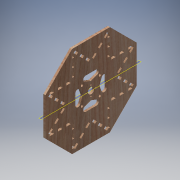
# Autodesk Inventor part: OctBase
Saved by Autodesk Inventor 2019 (Build 230136000, 136)
## iProperties
Created: 2019-01-14
Part Number: OctBase
Material: Wood (Birch)
Document SubType Name: Modeling
Designer: nxgam
Density: 0.55 g/cm^3
Appearance: Birch - Natural Polished
Author: nxgam
Autodesk Inventor part; units mm, degrees
ref_plane "YZ Plane" through (0, 0, 0) normal (1, 0, 0) x (0, 1, 0)
ref_plane "XZ Plane" through (0, 0, 0) normal (0, 1, 0) x (-1, 0, 0)
ref_plane "XY Plane" through (0, 0, 0) normal (0, 0, 1) x (1, 0, 0)
sketch "Sketch1" plane through (0, 0, 0) normal (1, 0, 0) x (0, 1, 0)
  line L0 (-110.3778, -45.72) -> (-110.3778, 45.72)
  line L1 (-110.3778, 45.72) -> (-45.72, 110.3778)
  line L2 (-45.72, 110.3778) -> (45.72, 110.3778)
  line L3 (45.72, 110.3778) -> (110.3778, 45.72)
  line L4 (110.3778, 45.72) -> (110.3778, -45.72)
  line L5 (110.3778, -45.72) -> (45.72, -110.3778)
  line L6 (45.72, -110.3778) -> (-45.72, -110.3778)
  line L7 (-45.72, -110.3778) -> (-110.3778, -45.72)
  point P0 (0, 0)
  point P1 (0, 0)
  dimension "d0" = 91.44
  constraints: 16 end point, 1 coincident, 1 horizontal, 17 other
  measures "d0" distance of L3.end L4.end
extrude "Extrusion1" add sketch "Sketch1" along normal blind 5.08
sketch "Sketch2" plane through (5.08, 0, 0) normal (1, 0, 0) x (0, 0, -1)
  line L0 (-45.72, 59.5778) -> (-40.64, 59.5778)
  line L1 (-40.64, 59.5778) -> (-40.64, 49.4178)
  line L2 (-40.64, 49.4178) -> (-45.72, 49.4178)
  line L3 (-45.72, 49.4178) -> (-45.72, 59.5778)
  line L4 (-45.72, 79.8978) -> (-40.64, 79.8978)
  line L5 (-40.64, 79.8978) -> (-40.64, 69.7378)
  line L6 (-40.64, 69.7378) -> (-45.72, 69.7378)
  line L7 (-45.72, 69.7378) -> (-45.72, 79.8978)
  line L8 (-45.72, 100.2178) -> (-40.64, 100.2178)
  line L9 (-40.64, 100.2178) -> (-40.64, 90.0578)
  line L10 (-40.64, 90.0578) -> (-45.72, 90.0578)
  line L11 (-45.72, 90.0578) -> (-45.72, 100.2178)
  line L12 (-40.64, 110.3778) -> (-45.72, 110.3778)
  line L13 (-45.72, 110.3778) -> (-45.72, 120.5378)
  line L14 (-45.72, 120.5378) -> (-40.64, 120.5378)
  line L15 (-40.64, 120.5378) -> (-40.64, 110.3778)
  line L16 (-45.72, 130.6978) -> (-45.72, 140.8578)
  line L17 (-45.72, 140.8578) -> (-40.64, 140.8578)
  line L18 (-40.64, 140.8578) -> (-40.64, 130.6978)
  line L19 (-40.64, 130.6978) -> (-45.72, 130.6978)
  line L20 (-45.72, 151.0178) -> (-45.72, 161.1778)
  line L21 (-45.72, 161.1778) -> (-40.64, 161.1778)
  line L22 (-40.64, 161.1778) -> (-40.64, 151.0178)
  line L23 (-40.64, 151.0178) -> (-45.72, 151.0178)
  line L24 (-45.72, 171.3378) -> (-45.72, 181.4978)
  line L25 (-45.72, 181.4978) -> (-40.64, 181.4978)
  line L26 (-40.64, 181.4978) -> (-40.64, 171.3378)
  line L27 (-40.64, 171.3378) -> (-45.72, 171.3378)
  line L28 (-45.72, 191.6578) -> (-45.72, 201.8178)
  line L29 (-45.72, 201.8178) -> (-40.64, 201.8178)
  line L30 (-40.64, 201.8178) -> (-40.64, 191.6578)
  line L31 (-40.64, 191.6578) -> (-45.72, 191.6578)
  line L32 (-45.72, 211.9778) -> (-45.72, 222.1378)
  line L33 (-45.72, 222.1378) -> (-40.64, 222.1378)
  line L34 (-40.64, 222.1378) -> (-40.64, 211.9778)
  line L35 (-40.64, 211.9778) -> (-45.72, 211.9778)
  line L36 (-45.72, 232.2978) -> (-45.72, 242.4578)
  line L37 (-45.72, 242.4578) -> (-40.64, 242.4578)
  line L38 (-40.64, 242.4578) -> (-40.64, 232.2978)
  line L39 (-40.64, 232.2978) -> (-45.72, 232.2978)
  line L40 (-45.72, 252.6178) -> (-45.72, 262.7778)
  line L41 (-45.72, 262.7778) -> (-40.64, 262.7778)
  line L42 (-40.64, 262.7778) -> (-40.64, 252.6178)
  line L43 (-40.64, 252.6178) -> (-45.72, 252.6178)
  line L44 (-45.72, 272.9378) -> (-45.72, 283.0978)
  line L45 (-45.72, 283.0978) -> (-40.64, 283.0978)
  line L46 (-40.64, 283.0978) -> (-40.64, 272.9378)
  line L47 (-40.64, 272.9378) -> (-45.72, 272.9378)
  line L48 (-45.72, 293.2578) -> (-45.72, 303.4178)
  line L49 (-45.72, 303.4178) -> (-40.64, 303.4178)
  line L50 (-40.64, 303.4178) -> (-40.64, 293.2578)
  line L51 (-40.64, 293.2578) -> (-45.72, 293.2578)
  line L52 (-45.72, 313.5778) -> (-45.72, 323.7378)
  line L53 (-45.72, 323.7378) -> (-40.64, 323.7378)
  line L54 (-40.64, 323.7378) -> (-40.64, 313.5778)
  line L55 (-40.64, 313.5778) -> (-45.72, 313.5778)
  line L56 (-45.72, 333.8978) -> (-45.72, 344.0578)
  line L57 (-45.72, 344.0578) -> (-40.64, 344.0578)
  line L58 (-40.64, 344.0578) -> (-40.64, 333.8978)
  line L59 (-40.64, 333.8978) -> (-45.72, 333.8978)
  line L60 (-45.72, 354.2178) -> (-45.72, 364.3778)
  line L61 (-45.72, 364.3778) -> (-40.64, 364.3778)
  line L62 (-40.64, 364.3778) -> (-40.64, 354.2178)
  line L63 (-40.64, 354.2178) -> (-45.72, 354.2178)
  line L64 (-45.72, 374.5378) -> (-45.72, 384.6978)
  line L65 (-45.72, 384.6978) -> (-40.64, 384.6978)
  line L66 (-40.64, 384.6978) -> (-40.64, 374.5378)
  line L67 (-40.64, 374.5378) -> (-45.72, 374.5378)
  line L68 (-45.72, 394.8578) -> (-45.72, 405.0178)
  line L69 (-45.72, 405.0178) -> (-40.64, 405.0178)
  line L70 (-40.64, 405.0178) -> (-40.64, 394.8578)
  line L71 (-40.64, 394.8578) -> (-45.72, 394.8578)
  line L72 (-45.72, 415.1778) -> (-45.72, 425.3378)
  line L73 (-45.72, 425.3378) -> (-40.64, 425.3378)
  line L74 (-40.64, 425.3378) -> (-40.64, 415.1778)
  line L75 (-40.64, 415.1778) -> (-45.72, 415.1778)
  line L76 (-45.72, 435.4978) -> (-45.72, 473.3735)
  line L77 (-45.72, 473.3735) -> (-40.64, 473.3735)
  line L78 (-40.64, 473.3735) -> (-40.64, 435.4978)
  line L79 (-40.64, 435.4978) -> (-45.72, 435.4978)
  line L80 (40.64, 59.5778) -> (45.72, 59.5778)
  line L81 (45.72, 59.5778) -> (45.72, 49.4178)
  line L82 (45.72, 49.4178) -> (40.64, 49.4178)
  line L83 (40.64, 49.4178) -> (40.64, 59.5778)
  line L84 (40.64, 79.8978) -> (45.72, 79.8978)
  line L85 (45.72, 79.8978) -> (45.72, 69.7378)
  line L86 (45.72, 69.7378) -> (40.64, 69.7378)
  line L87 (40.64, 69.7378) -> (40.64, 79.8978)
  line L88 (40.64, 100.2178) -> (45.72, 100.2178)
  line L89 (45.72, 100.2178) -> (45.72, 90.0578)
  line L90 (45.72, 90.0578) -> (40.64, 90.0578)
  line L91 (40.64, 90.0578) -> (40.64, 100.2178)
  line L92 (45.72, 110.3778) -> (40.64, 110.3778)
  line L93 (40.64, 110.3778) -> (40.64, 120.5378)
  line L94 (40.64, 120.5378) -> (45.72, 120.5378)
  line L95 (45.72, 120.5378) -> (45.72, 110.3778)
  line L96 (40.64, 130.6978) -> (40.64, 140.8578)
  line L97 (40.64, 140.8578) -> (45.72, 140.8578)
  line L98 (45.72, 140.8578) -> (45.72, 130.6978)
  line L99 (45.72, 130.6978) -> (40.64, 130.6978)
  line L100 (40.64, 151.0178) -> (40.64, 161.1778)
  line L101 (40.64, 161.1778) -> (45.72, 161.1778)
  line L102 (45.72, 161.1778) -> (45.72, 151.0178)
  line L103 (45.72, 151.0178) -> (40.64, 151.0178)
  line L104 (40.64, 171.3378) -> (40.64, 181.4978)
  line L105 (40.64, 181.4978) -> (45.72, 181.4978)
  line L106 (45.72, 181.4978) -> (45.72, 171.3378)
  line L107 (45.72, 171.3378) -> (40.64, 171.3378)
  line L108 (40.64, 191.6578) -> (40.64, 201.8178)
  line L109 (40.64, 201.8178) -> (45.72, 201.8178)
  line L110 (45.72, 201.8178) -> (45.72, 191.6578)
  line L111 (45.72, 191.6578) -> (40.64, 191.6578)
  line L112 (40.64, 211.9778) -> (40.64, 222.1378)
  line L113 (40.64, 222.1378) -> (45.72, 222.1378)
  line L114 (45.72, 222.1378) -> (45.72, 211.9778)
  line L115 (45.72, 211.9778) -> (40.64, 211.9778)
  line L116 (40.64, 232.2978) -> (40.64, 242.4578)
  line L117 (40.64, 242.4578) -> (45.72, 242.4578)
  line L118 (45.72, 242.4578) -> (45.72, 232.2978)
  line L119 (45.72, 232.2978) -> (40.64, 232.2978)
  line L120 (40.64, 252.6178) -> (40.64, 262.7778)
  line L121 (40.64, 262.7778) -> (45.72, 262.7778)
  line L122 (45.72, 262.7778) -> (45.72, 252.6178)
  line L123 (45.72, 252.6178) -> (40.64, 252.6178)
  line L124 (40.64, 272.9378) -> (40.64, 283.0978)
  line L125 (40.64, 283.0978) -> (45.72, 283.0978)
  line L126 (45.72, 283.0978) -> (45.72, 272.9378)
  line L127 (45.72, 272.9378) -> (40.64, 272.9378)
  line L128 (40.64, 293.2578) -> (40.64, 303.4178)
  line L129 (40.64, 303.4178) -> (45.72, 303.4178)
  line L130 (45.72, 303.4178) -> (45.72, 293.2578)
  line L131 (45.72, 293.2578) -> (40.64, 293.2578)
  line L132 (40.64, 313.5778) -> (40.64, 323.7378)
  line L133 (40.64, 323.7378) -> (45.72, 323.7378)
  line L134 (45.72, 323.7378) -> (45.72, 313.5778)
  line L135 (45.72, 313.5778) -> (40.64, 313.5778)
  line L136 (40.64, 333.8978) -> (40.64, 344.0578)
  line L137 (40.64, 344.0578) -> (45.72, 344.0578)
  line L138 (45.72, 344.0578) -> (45.72, 333.8978)
  line L139 (45.72, 333.8978) -> (40.64, 333.8978)
  line L140 (40.64, 354.2178) -> (40.64, 364.3778)
  line L141 (40.64, 364.3778) -> (45.72, 364.3778)
  line L142 (45.72, 364.3778) -> (45.72, 354.2178)
  line L143 (45.72, 354.2178) -> (40.64, 354.2178)
  line L144 (40.64, 374.5378) -> (40.64, 384.6978)
  line L145 (40.64, 384.6978) -> (45.72, 384.6978)
  line L146 (45.72, 384.6978) -> (45.72, 374.5378)
  line L147 (45.72, 374.5378) -> (40.64, 374.5378)
  line L148 (40.64, 394.8578) -> (40.64, 405.0178)
  line L149 (40.64, 405.0178) -> (45.72, 405.0178)
  line L150 (45.72, 405.0178) -> (45.72, 394.8578)
  line L151 (45.72, 394.8578) -> (40.64, 394.8578)
  line L152 (40.64, 415.1778) -> (40.64, 425.3378)
  line L153 (40.64, 425.3378) -> (45.72, 425.3378)
  line L154 (45.72, 425.3378) -> (45.72, 415.1778)
  line L155 (45.72, 415.1778) -> (40.64, 415.1778)
  line L156 (40.64, 435.4978) -> (40.64, 473.3735)
  line L157 (40.64, 473.3735) -> (45.72, 473.3735)
  line L158 (45.72, 473.3735) -> (45.72, 435.4978)
  line L159 (45.72, 435.4978) -> (40.64, 435.4978)
  line L160 (-103.1936, 38.5358) -> (-99.6015, 42.1279)
  line L161 (-92.4173, 34.9437) -> (-96.0094, 31.3516)
  line L162 (-96.0094, 31.3516) -> (-103.1936, 38.5358)
  line L163 (-88.8252, 24.1674) -> (-85.2331, 27.7595)
  line L164 (-85.2331, 27.7595) -> (-78.0489, 20.5753)
  line L165 (-78.0489, 20.5753) -> (-81.641, 16.9832)
  line L166 (-81.641, 16.9832) -> (-88.8252, 24.1674)
  line L167 (-74.4568, 9.799) -> (-70.8647, 13.3911)
  line L168 (-70.8647, 13.3911) -> (-63.6805, 6.2069)
  line L169 (-63.6805, 6.2069) -> (-67.2726, 2.6148)
  line L170 (-67.2726, 2.6148) -> (-74.4568, 9.799)
  line L171 (-99.6015, 42.1279) -> (-92.4173, 34.9437)
  line L172 (-42.1279, 99.6015) -> (-38.5358, 103.1936)
  line L173 (-38.5358, 103.1936) -> (-31.3516, 96.0094)
  line L174 (-34.9437, 92.4173) -> (-42.1279, 99.6015)
  line L175 (-31.3516, 96.0094) -> (-34.9437, 92.4173)
  line L176 (-27.7595, 85.2331) -> (-24.1674, 88.8252)
  line L177 (-20.5753, 78.0489) -> (-27.7595, 85.2331)
  line L178 (-16.9832, 81.641) -> (-20.5753, 78.0489)
  line L179 (-13.3911, 70.8647) -> (-9.799, 74.4568)
  line L180 (-6.2069, 63.6805) -> (-13.3911, 70.8647)
  line L181 (-2.6148, 67.2726) -> (-6.2069, 63.6805)
  line L182 (-9.799, 74.4568) -> (-2.6148, 67.2726)
  line L183 (-24.1674, 88.8252) -> (-16.9832, 81.641)
  line L184 (-100.2178, -45.72) -> (-100.2178, -40.64)
  line L185 (-90.0578, -40.64) -> (-90.0578, -45.72)
  line L186 (-90.0578, -45.72) -> (-100.2178, -45.72)
  line L187 (-79.8978, -45.72) -> (-79.8978, -40.64)
  line L188 (-79.8978, -40.64) -> (-69.7378, -40.64)
  line L189 (-69.7378, -40.64) -> (-69.7378, -45.72)
  line L190 (-69.7378, -45.72) -> (-79.8978, -45.72)
  line L191 (-59.5778, -45.72) -> (-59.5778, -40.64)
  line L192 (-59.5778, -40.64) -> (-49.4178, -40.64)
  line L193 (-49.4178, -40.64) -> (-49.4178, -45.72)
  line L194 (-49.4178, -45.72) -> (-59.5778, -45.72)
  line L195 (-100.2178, -40.64) -> (-90.0578, -40.64)
  line L196 (-100.2178, 40.64) -> (-100.2178, 45.72)
  line L197 (-100.2178, 45.72) -> (-90.0578, 45.72)
  line L198 (-90.0578, 40.64) -> (-100.2178, 40.64)
  line L199 (-90.0578, 45.72) -> (-90.0578, 40.64)
  line L200 (-79.8978, 40.64) -> (-79.8978, 45.72)
  line L201 (-69.7378, 40.64) -> (-79.8978, 40.64)
  line L202 (-69.7378, 45.72) -> (-69.7378, 40.64)
  line L203 (-59.5778, 40.64) -> (-59.5778, 45.72)
  line L204 (-49.4178, 40.64) -> (-59.5778, 40.64)
  line L205 (-49.4178, 45.72) -> (-49.4178, 40.64)
  line L206 (-59.5778, 45.72) -> (-49.4178, 45.72)
  line L207 (-79.8978, 45.72) -> (-69.7378, 45.72)
  line L208 (-38.5358, -103.1936) -> (-42.1279, -99.6015)
  line L209 (-34.9437, -92.4173) -> (-31.3516, -96.0094)
  line L210 (-31.3516, -96.0094) -> (-38.5358, -103.1936)
  line L211 (-24.1674, -88.8252) -> (-27.7595, -85.2331)
  line L212 (-27.7595, -85.2331) -> (-20.5753, -78.0489)
  line L213 (-20.5753, -78.0489) -> (-16.9832, -81.641)
  line L214 (-16.9832, -81.641) -> (-24.1674, -88.8252)
  line L215 (-9.799, -74.4568) -> (-13.3911, -70.8647)
  line L216 (-13.3911, -70.8647) -> (-6.2069, -63.6805)
  line L217 (-6.2069, -63.6805) -> (-2.6148, -67.2726)
  line L218 (-2.6148, -67.2726) -> (-9.799, -74.4568)
  line L219 (-42.1279, -99.6015) -> (-34.9437, -92.4173)
  line L220 (-99.6015, -42.1279) -> (-103.1936, -38.5358)
  line L221 (-103.1936, -38.5358) -> (-96.0094, -31.3516)
  line L222 (-92.4173, -34.9437) -> (-99.6015, -42.1279)
  line L223 (-96.0094, -31.3516) -> (-92.4173, -34.9437)
  line L224 (-85.2331, -27.7595) -> (-88.8252, -24.1674)
  line L225 (-78.0489, -20.5753) -> (-85.2331, -27.7595)
  line L226 (-81.641, -16.9832) -> (-78.0489, -20.5753)
  line L227 (-70.8647, -13.3911) -> (-74.4568, -9.799)
  line L228 (-63.6805, -6.2069) -> (-70.8647, -13.3911)
  line L229 (-67.2726, -2.6148) -> (-63.6805, -6.2069)
  line L230 (-74.4568, -9.799) -> (-67.2726, -2.6148)
  line L231 (-88.8252, -24.1674) -> (-81.641, -16.9832)
  line L232 (45.72, -100.2178) -> (40.64, -100.2178)
  line L233 (40.64, -90.0578) -> (45.72, -90.0578)
  line L234 (45.72, -90.0578) -> (45.72, -100.2178)
  line L235 (45.72, -79.8978) -> (40.64, -79.8978)
  line L236 (40.64, -79.8978) -> (40.64, -69.7378)
  line L237 (40.64, -69.7378) -> (45.72, -69.7378)
  line L238 (45.72, -69.7378) -> (45.72, -79.8978)
  line L239 (45.72, -59.5778) -> (40.64, -59.5778)
  line L240 (40.64, -59.5778) -> (40.64, -49.4178)
  line L241 (40.64, -49.4178) -> (45.72, -49.4178)
  line L242 (45.72, -49.4178) -> (45.72, -59.5778)
  line L243 (40.64, -100.2178) -> (40.64, -90.0578)
  line L244 (-40.64, -100.2178) -> (-45.72, -100.2178)
  line L245 (-45.72, -100.2178) -> (-45.72, -90.0578)
  line L246 (-40.64, -90.0578) -> (-40.64, -100.2178)
  line L247 (-45.72, -90.0578) -> (-40.64, -90.0578)
  line L248 (-40.64, -79.8978) -> (-45.72, -79.8978)
  line L249 (-40.64, -69.7378) -> (-40.64, -79.8978)
  line L250 (-45.72, -69.7378) -> (-40.64, -69.7378)
  line L251 (-40.64, -59.5778) -> (-45.72, -59.5778)
  line L252 (-40.64, -49.4178) -> (-40.64, -59.5778)
  line L253 (-45.72, -49.4178) -> (-40.64, -49.4178)
  line L254 (-45.72, -59.5778) -> (-45.72, -49.4178)
  line L255 (-45.72, -79.8978) -> (-45.72, -69.7378)
  line L256 (103.1936, -38.5358) -> (99.6015, -42.1279)
  line L257 (92.4173, -34.9437) -> (96.0094, -31.3516)
  line L258 (96.0094, -31.3516) -> (103.1936, -38.5358)
  line L259 (88.8252, -24.1674) -> (85.2331, -27.7595)
  line L260 (85.2331, -27.7595) -> (78.0489, -20.5753)
  line L261 (78.0489, -20.5753) -> (81.641, -16.9832)
  line L262 (81.641, -16.9832) -> (88.8252, -24.1674)
  line L263 (74.4568, -9.799) -> (70.8647, -13.3911)
  line L264 (70.8647, -13.3911) -> (63.6805, -6.2069)
  line L265 (63.6805, -6.2069) -> (67.2726, -2.6148)
  line L266 (67.2726, -2.6148) -> (74.4568, -9.799)
  line L267 (99.6015, -42.1279) -> (92.4173, -34.9437)
  line L268 (42.1279, -99.6015) -> (38.5358, -103.1936)
  line L269 (38.5358, -103.1936) -> (31.3516, -96.0094)
  line L270 (34.9437, -92.4173) -> (42.1279, -99.6015)
  line L271 (31.3516, -96.0094) -> (34.9437, -92.4173)
  line L272 (27.7595, -85.2331) -> (24.1674, -88.8252)
  line L273 (20.5753, -78.0489) -> (27.7595, -85.2331)
  line L274 (16.9832, -81.641) -> (20.5753, -78.0489)
  line L275 (13.3911, -70.8647) -> (9.799, -74.4568)
  line L276 (6.2069, -63.6805) -> (13.3911, -70.8647)
  line L277 (2.6148, -67.2726) -> (6.2069, -63.6805)
  line L278 (9.799, -74.4568) -> (2.6148, -67.2726)
  line L279 (24.1674, -88.8252) -> (16.9832, -81.641)
  line L280 (100.2178, 45.72) -> (100.2178, 40.64)
  line L281 (90.0578, 40.64) -> (90.0578, 45.72)
  line L282 (90.0578, 45.72) -> (100.2178, 45.72)
  line L283 (79.8978, 45.72) -> (79.8978, 40.64)
  line L284 (79.8978, 40.64) -> (69.7378, 40.64)
  line L285 (69.7378, 40.64) -> (69.7378, 45.72)
  line L286 (69.7378, 45.72) -> (79.8978, 45.72)
  line L287 (59.5778, 45.72) -> (59.5778, 40.64)
  line L288 (59.5778, 40.64) -> (49.4178, 40.64)
  line L289 (49.4178, 40.64) -> (49.4178, 45.72)
  line L290 (49.4178, 45.72) -> (59.5778, 45.72)
  line L291 (100.2178, 40.64) -> (90.0578, 40.64)
  line L292 (100.2178, -40.64) -> (100.2178, -45.72)
  line L293 (100.2178, -45.72) -> (90.0578, -45.72)
  line L294 (90.0578, -40.64) -> (100.2178, -40.64)
  line L295 (90.0578, -45.72) -> (90.0578, -40.64)
  line L296 (79.8978, -40.64) -> (79.8978, -45.72)
  line L297 (69.7378, -40.64) -> (79.8978, -40.64)
  line L298 (69.7378, -45.72) -> (69.7378, -40.64)
  line L299 (59.5778, -40.64) -> (59.5778, -45.72)
  line L300 (49.4178, -40.64) -> (59.5778, -40.64)
  line L301 (49.4178, -45.72) -> (49.4178, -40.64)
  line L302 (59.5778, -45.72) -> (49.4178, -45.72)
  line L303 (79.8978, -45.72) -> (69.7378, -45.72)
  line L304 (38.5358, 103.1936) -> (42.1279, 99.6015)
  line L305 (34.9437, 92.4173) -> (31.3516, 96.0094)
  line L306 (31.3516, 96.0094) -> (38.5358, 103.1936)
  line L307 (24.1674, 88.8252) -> (27.7595, 85.2331)
  line L308 (27.7595, 85.2331) -> (20.5753, 78.0489)
  line L309 (20.5753, 78.0489) -> (16.9832, 81.641)
  line L310 (16.9832, 81.641) -> (24.1674, 88.8252)
  line L311 (9.799, 74.4568) -> (13.3911, 70.8647)
  line L312 (13.3911, 70.8647) -> (6.2069, 63.6805)
  line L313 (6.2069, 63.6805) -> (2.6148, 67.2726)
  line L314 (2.6148, 67.2726) -> (9.799, 74.4568)
  line L315 (42.1279, 99.6015) -> (34.9437, 92.4173)
  line L316 (99.6015, 42.1279) -> (103.1936, 38.5358)
  line L317 (103.1936, 38.5358) -> (96.0094, 31.3516)
  line L318 (92.4173, 34.9437) -> (99.6015, 42.1279)
  line L319 (96.0094, 31.3516) -> (92.4173, 34.9437)
  line L320 (85.2331, 27.7595) -> (88.8252, 24.1674)
  line L321 (78.0489, 20.5753) -> (85.2331, 27.7595)
  line L322 (81.641, 16.9832) -> (78.0489, 20.5753)
  line L323 (70.8647, 13.3911) -> (74.4568, 9.799)
  line L324 (63.6805, 6.2069) -> (70.8647, 13.3911)
  line L325 (67.2726, 2.6148) -> (63.6805, 6.2069)
  line L326 (74.4568, 9.799) -> (67.2726, 2.6148)
  line L327 (88.8252, 24.1674) -> (81.641, 16.9832)
  line L328 (-45.72, -110.3778) -> (45.72, -110.3778) projected
  line L329 (45.72, -110.3778) -> (110.3778, -45.72) projected
  line L330 (110.3778, -45.72) -> (110.3778, 45.72) projected
  line L331 (110.3778, 45.72) -> (45.72, 110.3778) projected
  line L332 (45.72, 110.3778) -> (-45.72, 110.3778) projected
  line L333 (-45.72, 110.3778) -> (-110.3778, 45.72) projected
  line L334 (-110.3778, 45.72) -> (-110.3778, -45.72) projected
  line L335 (-110.3778, -45.72) -> (-45.72, -110.3778) projected
  point P0 (0, 0)
  dimension "d5" = 360
  constraints: 656 end point, 80 horizontal, 80 vertical, 545 other
extrude "Extrusion2" cut sketch "Sketch2" against normal blind 25.4 contours L332 L92 L331 L330 L329 L328 L335 L334 L333 L12 keep common part
sketch "Sketch4" plane through (5.08, 0, 0) normal (1, 0, 0) x (0, 0, -1)
  circle A0 centre (0, 0) radius 7.62
  dimension "d9" = 15.24
  constraints: 1 centre point, 1 coincident
  measures "d9" diameter of A0
extrude "Extrusion3" cut sketch "Sketch4" against normal blind 25.4
sketch "Sketch5" plane through (5.08, 0, 0) normal (1, 0, 0) x (0, 0, -1)
  line L0 (31.75, 12.7) -> (31.75, -12.7) construction
  line L1 (25.4, 12.7) -> (25.4, -12.7) construction
  line L2 (38.1, -12.7) -> (38.1, 12.7)
  arc A0 (38.1, 12.7) -> (25.4, 12.7) centre (31.75, 12.7) ccw
  arc A1 (25.4, -12.7) -> (38.1, -12.7) centre (31.75, -12.7) ccw
  line L3 (0, 0) -> (110.3778, 0) construction
  line L4 (110.3778, 45.72) -> (110.3778, -45.72) construction
  line L5 (25.7894, -14.8895) -> (20.7221, -1.0948)
  line L6 (25.7894, 14.8895) -> (20.7221, 1.0948)
  arc A2 (20.7221, 1.0948) -> (20.7221, -1.0948) centre (23.7024, 0) ccw
  line L7 (-12.7, 31.75) -> (12.7, 31.75) construction
  line L8 (-12.7, 25.4) -> (12.7, 25.4) construction
  line L9 (12.7, 38.1) -> (-12.7, 38.1)
  arc A3 (-12.7, 38.1) -> (-12.7, 25.4) centre (-12.7, 31.75) ccw
  arc A4 (12.7, 25.4) -> (12.7, 38.1) centre (12.7, 31.75) ccw
  line L10 (14.8895, 25.7894) -> (1.0948, 20.7221)
  line L11 (-14.8895, 25.7894) -> (-1.0948, 20.7221)
  arc A5 (-1.0948, 20.7221) -> (1.0948, 20.7221) centre (0, 23.7024) ccw
  line L12 (-31.75, -12.7) -> (-31.75, 12.7) construction
  line L13 (-25.4, -12.7) -> (-25.4, 12.7) construction
  line L14 (-38.1, 12.7) -> (-38.1, -12.7)
  arc A6 (-38.1, -12.7) -> (-25.4, -12.7) centre (-31.75, -12.7) ccw
  arc A7 (-25.4, 12.7) -> (-38.1, 12.7) centre (-31.75, 12.7) ccw
  line L15 (-25.7894, 14.8895) -> (-20.7221, 1.0948)
  line L16 (-25.7894, -14.8895) -> (-20.7221, -1.0948)
  arc A8 (-20.7221, -1.0948) -> (-20.7221, 1.0948) centre (-23.7024, 0) ccw
  line L17 (12.7, -31.75) -> (-12.7, -31.75) construction
  line L18 (12.7, -25.4) -> (-12.7, -25.4) construction
  line L19 (-12.7, -38.1) -> (12.7, -38.1)
  arc A9 (12.7, -38.1) -> (12.7, -25.4) centre (12.7, -31.75) ccw
  arc A10 (-12.7, -25.4) -> (-12.7, -38.1) centre (-12.7, -31.75) ccw
  line L20 (-14.8895, -25.7894) -> (-1.0948, -20.7221)
  line L21 (14.8895, -25.7894) -> (1.0948, -20.7221)
  arc A11 (1.0948, -20.7221) -> (-1.0948, -20.7221) centre (0, -23.7024) ccw
  point P0 (31.75, 0)
  point P1 (20.32, 0)
  point P2 (0, 31.75)
  point P3 (0, 20.32)
  point P4 (-31.75, 0)
  point P5 (-20.32, 0)
  point P6 (0, -31.75)
  point P7 (0, -20.32)
  dimension "d13" = 31.75
  dimension "d14" = 25.4
  dimension "d30" = 6.35
  dimension "d31" = 5.08
  dimension "d32" = 3.175
  dimension "d35" = 360
  constraints: 50 end point, 32 point on circle, 12 centre point, 10 point on line, 8 tangent, 2 midpoint, 1 parallel, 1 vertical, 85 other
  measures "d13" distance from line of L0 L3.start
  measures "d14" distance of L0.start L0.end
  measures "d30" radius of A1
  measures "d31" distance from line of point (20.32, 0) L1
  measures "d32" radius of A2
extrude "Extrusion4" cut sketch "Sketch5" against normal blind 25.4
sketch "Sketch6" plane through (5.08, 0, 0) normal (1, 0, 0) x (0, 0, -1)
  circle A0 centre (-11.938, 0) radius 1.5 projected
  circle A1 centre (11.938, 0) radius 1.5 projected
  circle A2 centre (0, -11.938) radius 1.5 projected
  circle A3 centre (0, 11.938) radius 1.5 projected
  circle A4 centre (0, 0) radius 6 projected
  circle A5 centre (0, 0) radius 16 projected
  point P0 (0, 0)
  constraints: 4 coincident
hole "Hole1" at (5.08, 11.938, 0) at (5.08, 0, -11.938) at (5.08, -11.938, 0) at (5.08, 0, 11.938) direction (-1, 0, 0) diameter 3 end through all
ref_plane "Work Plane1" through (0, 0, -45.72) normal (0, -1, 0) x (1, 0, 0)
sketch "Sketch8" plane through (0, 0, 0) normal (-1, 0, 0) x (0, 0, 1)
  arc A0 (-19.6668, -23.7977) -> (-23.7977, -19.6668) centre (-21.7322, -21.7322) ccw
  circle A1 centre (-21.7322, -21.7322) radius 3
  point P0 (0, 0)
  dimension "d37" = 6
  constraints: 2 centre point, 2 point on circle, 1 coincident, 4 other
  measures "d37" diameter of A1
extrude "Extrusion5" cut sketch "Sketch8" against normal blind 25.4
pattern_circular "Circular Pattern1" count 4 over 360 about axis through (5.08, 0, 0) along (-1, 0, 0) of "Extrusion5"
body "Solid1"
